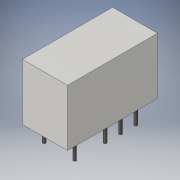
# Autodesk Inventor part: EC2-5NU_Relay
Saved by Autodesk Inventor 2016 (Build 200138000, 138)
## iProperties
Created: 2016-09-10
Part Number: EC2-5NU_Relay
Material: Generic
Document SubType Name: Modeling
Designer: jfixelle
Density: 1 g/cm^3
Appearance: White
Author: jfixelle
Autodesk Inventor part; units mm, degrees
ref_plane "YZ Plane" through (0, 0, 0) normal (1, 0, 0) x (0, 1, 0)
ref_plane "XZ Plane" through (0, 0, 0) normal (0, 1, 0) x (-1, 0, 0)
ref_plane "XY Plane" through (0, 0, 0) normal (0, 0, 1) x (1, 0, 0)
sketch "Sketch1" plane through (0, 0, 0) normal (0, 1, 0) x (-1, 0, 0)
  line L0 (3.75, 7.5) -> (-3.75, 7.5)
  line L1 (-3.75, 7.5) -> (-3.75, -7.5)
  line L2 (-3.75, -7.5) -> (3.75, -7.5)
  line L3 (3.75, -7.5) -> (3.75, 7.5)
  point P0 (0, 0)
  dimension "d0" = 15
  dimension "d1" = 7.5
  dimension "d2" = 7.5
  dimension "d3" = 3.75
  constraints: 8 end point, 2 parallel, 1 horizontal, 1 perpendicular
  measures "d0" distance of L2.end L0.start
  measures "d1" distance from line of point (0, 0) L2
  measures "d2" distance of L1.end L2.end
  measures "d3" distance from line of point (0, 0) L3
extrude "Extrusion1" add sketch "Sketch1" along normal blind 9.4
sketch "Sketch2" plane through (0, 0, 0) normal (0, -1, 0) x (1, 0, 0)
  circle A0 centre (2.54, 5.08) radius 0.25
  line L0 (0, 0) -> (0, -1.471)
  circle A1 centre (2.54, 2.54) radius 0.25
  circle A2 centre (2.54, 0) radius 0.25
  circle A3 centre (2.54, -2.54) radius 0.25
  circle A4 centre (2.54, -5.08) radius 0.25
  circle A5 centre (-2.54, 5.08) radius 0.25
  circle A6 centre (-2.54, 2.54) radius 0.25
  circle A7 centre (-2.54, 0) radius 0.25
  circle A8 centre (-2.54, -2.54) radius 0.25
  circle A9 centre (-2.54, -5.08) radius 0.25
  dimension "d6" = 5.08
  dimension "d7" = 2.54
  dimension "d8" = 0.5
  dimension "d11" = 2.54
  constraints: 10 centre point, 5 symmetric about line, 2 end point, 2 vertical, 13 other
  measures "d6" vertical distance of L0.start A0.centre
  measures "d7" horizontal distance of L0.start A0.centre
  measures "d8" diameter of A0
  measures "d11" distance of A0.centre A1.centre
extrude "Extrusion2" add sketch "Sketch2" along normal blind 3.2 contours A0 | A2 | A3 | A4 | A5 | A7 | A8 | A9
body "Solid1"
